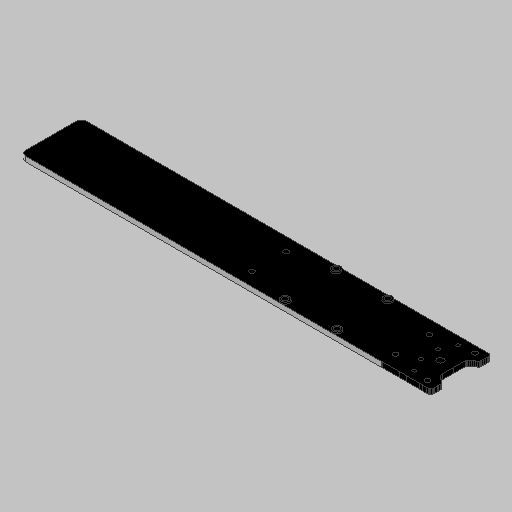
# Autodesk Inventor part: Part3
Saved by Autodesk Inventor 2025.2 (Build 292293000, 293)
## iProperties
Created: 2025-03-10
Part Number: Part3
Material: Generic
Document SubType Name: Modeling
Designer: joaki
Density: 1 g/cm^3
Appearance: Default
Author: joaki
Autodesk Inventor part; units mm, degrees
(part 1 of 5)
ref_plane "YZ Plane" through (0, 0, 0) normal (1, 0, 0) x (0, 1, 0)
ref_plane "XZ Plane" through (0, 0, 0) normal (0, 1, 0) x (-1, 0, 0)
ref_plane "XY Plane" through (0, 0, 0) normal (0, 0, 1) x (1, 0, 0)
sketch "Sketch1" plane through (0, 0, 0) normal (0, 1, 0) x (-1, 0, 0)
  arc A0 (-32.0458, 49.1475) -> (-32.3532, 49.036) centre (-31.3396, 46.7212) ccw
  arc A1 (-32.3532, 49.036) -> (-32.6918, 48.8703) centre (-30.5708, 44.9654) ccw
  arc A2 (-32.6918, 48.8703) -> (-33.0092, 48.6799) centre (-30.623, 45.0615) ccw
  arc A3 (-33.0092, 48.6799) -> (-33.2503, 48.4933) centre (-31.9001, 46.9981) ccw
  arc A4 (-33.2503, 48.4933) -> (-33.966, 47.6322) centre (-30.6139, 45.5739) ccw
  arc A5 (-33.966, 47.6322) -> (-35.7265, 44.7103) centre (138.8211, -58.464) ccw
  arc A6 (-35.7265, 44.7103) -> (-37.4503, 41.7415) centre (154.4036, -67.6751) ccw
  arc A7 (-37.4503, 41.7415) -> (-37.8104, 40.7786) centre (-34.6555, 40.1476) ccw
  arc A8 (-37.8104, 40.7786) -> (-37.8194, 40.2827) centre (-36.4462, 40.5057) ccw
  arc A9 (-37.8194, 40.2827) -> (-37.3843, 37.657) centre (368.8514, 106.3279) ccw
  arc A10 (-37.3843, 37.657) -> (-36.8416, 34.5948) centre (155.765, 70.3074) ccw
  arc A11 (-36.8416, 34.5948) -> (-36.1725, 31.0888) centre (296.5053, 96.4035) ccw
  arc A12 (-35.5034, 27.5915) -> (-36.1725, 31.0888) centre (-396.5345, -39.6615) ccw
  arc A13 (-34.9615, 24.557) -> (-35.5034, 27.5915) centre (-238.8908, -10.2959) ccw
  arc A14 (-34.5206, 21.9365) -> (-34.9615, 24.557) centre (-543.7583, -62.3998) ccw
  arc A15 (-34.5375, 21.5226) -> (-34.5206, 21.9365) centre (-35.5244, 21.7703) ccw
  arc A16 (-34.665, 21.2419) -> (-34.5375, 21.5226) centre (-35.3707, 21.7317) ccw
  arc A17 (-34.9963, 20.7996) -> (-34.665, 21.2419) centre (-40.9474, 25.6026) ccw
  arc A18 (-35.4254, 20.3066) -> (-34.9963, 20.7996) centre (-41.848, 26.3295) ccw
  arc A19 (-35.9077, 19.8249) -> (-35.4254, 20.3066) centre (-43.0211, 27.4297) ccw
  line L0 (-35.9077, 19.8249) -> (-37.1415, 18.6708)
  line L1 (-37.1415, 18.6708) -> (-50.9288, 18.6708)
  line L2 (-50.9288, 18.6708) -> (-64.716, 18.6708)
  line L3 (-64.716, 18.6708) -> (-65.4406, 17.9462)
  arc A20 (-65.4406, 17.9462) -> (-65.8665, 17.4366) centre (-62.8082, 15.3139) ccw
  arc A21 (-65.8665, 17.4366) -> (-66.0686, 16.973) centre (-64.7983, 16.6952) ccw
  arc A22 (-66.0686, 16.973) -> (-66.1492, 16.2892) centre (-62.6302, 16.221) ccw
  arc A23 (-66.1492, 16.2892) -> (-66.1652, 14.6332) centre (19.2549, 14.6332) ccw
  arc A24 (-66.1652, 14.6332) -> (-66.0935, 12.6637) centre (-39.0795, 14.6332) ccw
  arc A25 (-66.0935, 12.6637) -> (-65.8047, 11.6707) centre (-63.6234, 12.8438) ccw
  arc A26 (-65.8047, 11.6707) -> (-65.1416, 10.9064) centre (-63.7738, 12.7629) ccw
  arc A27 (-65.1416, 10.9064) -> (-63.6042, 9.8709) centre (-52.1239, 28.5747) ccw
  arc A28 (-62.9662, 9.4495) -> (-63.6042, 9.8709) centre (-69.6262, 0.0598) ccw
  arc A29 (-62.3849, 9.0034) -> (-62.9662, 9.4495) centre (-68.5849, 1.5279) ccw
  arc A30 (-61.9232, 8.5909) -> (-62.3849, 9.0034) centre (-67.7613, 2.5209) ccw
  arc A31 (-61.7221, 8.31) -> (-61.9232, 8.5909) centre (-62.5797, 7.9083) ccw
  arc A32 (-61.4522, 7.1095) -> (-61.7221, 8.31) centre (-64.311, 7.0975) ccw
  arc A33 (-61.449, 0.3443) -> (-61.4522, 7.1095) centre (-966.3811, 3.2944) ccw
  arc A34 (-61.4895, -6.5686) -> (-61.449, 0.3443) centre (-1389.8333, 4.6747) ccw
  arc A35 (-61.7732, -7.3571) -> (-61.4895, -6.5686) centre (-62.7573, -6.5578) ccw
  arc A36 (-61.9835, -7.5631) -> (-61.7732, -7.3571) centre (-62.7825, -6.5373) ccw
  arc A37 (-62.517, -7.9679) -> (-61.9835, -7.5631) centre (-78.0906, 13.1153) ccw
  arc A38 (-63.1677, -8.4333) -> (-62.517, -7.9679) centre (-77.9814, 12.9674) ccw
  arc A39 (-63.8815, -8.9144) -> (-63.1677, -8.4333) centre (-83.0238, 20.252) ccw
  arc A40 (-63.8815, -8.9144) -> (-64.619, -9.4313) centre (-55.7825, -21.2545) ccw
  arc A41 (-64.619, -9.4313) -> (-65.2474, -9.9433) centre (-58.8117, -17.2015) ccw
  arc A42 (-65.2474, -9.9433) -> (-65.7227, -10.4032) centre (-60.2081, -15.6266) ccw
  arc A43 (-65.7227, -10.4032) -> (-65.9266, -10.7277) centre (-65.0137, -11.0748) ccw
  arc A44 (-65.9266, -10.7277) -> (-66.0195, -11.1058) centre (-64.4333, -11.2955) ccw
  arc A45 (-66.0195, -11.1058) -> (-66.0951, -11.8637) centre (-46.7413, -13.4108) ccw
  arc A46 (-66.0951, -11.8637) -> (-66.1477, -12.7646) centre (-45.1165, -13.5407) ccw
  arc A47 (-66.1477, -12.7646) -> (-66.1652, -13.7133) centre (-40.4419, -13.7133) ccw
  arc A48 (-66.1652, -13.7133) -> (-66.1479, -15.1982) centre (-2.5179, -13.7133) ccw
  arc A49 (-66.1479, -15.1982) -> (-66.0652, -15.8456) centre (-62.9983, -15.1247) ccw
  arc A50 (-66.0652, -15.8456) -> (-65.8627, -16.2951) centre (-64.8098, -15.5505) ccw
  arc A51 (-65.8627, -16.2951) -> (-65.4406, -16.7957) centre (-62.7118, -14.0669) ccw
  line L4 (-65.4406, -16.7957) -> (-64.716, -17.5203)
  line L5 (-64.716, -17.5203) -> (-50.9288, -17.5203)
  line L6 (-50.9288, -17.5203) -> (-37.1415, -17.5203)
  line L7 (-37.1415, -17.5203) -> (-35.9077, -18.6744)
  arc A52 (-35.4252, -19.1571) -> (-35.9077, -18.6744) centre (-42.8603, -26.1072) ccw
  arc A53 (-34.9953, -19.6532) -> (-35.4252, -19.1571) centre (-41.7875, -25.1044) ccw
  arc A54 (-34.6634, -20.0994) -> (-34.9953, -19.6532) centre (-40.8736, -24.3709) ccw
  arc A55 (-34.534, -20.386) -> (-34.6634, -20.0994) centre (-35.3938, -20.6018) ccw
  arc A56 (-34.5166, -20.8095) -> (-34.534, -20.386) centre (-35.5445, -20.6396) ccw
  arc A57 (-34.9565, -23.4263) -> (-34.5166, -20.8095) centre (-518.611, 59.2131) ccw
  arc A58 (-35.4987, -26.4597) -> (-34.9565, -23.4263) centre (-233.6422, 10.5217) ccw
  arc A59 (-36.1687, -29.953) -> (-35.4987, -26.4597) centre (-386.2783, 39.0092) ccw
  arc A60 (-36.1687, -29.953) -> (-36.8391, -33.4539) centre (295.6451, -95.311) ccw
  arc A61 (-36.8391, -33.4539) -> (-37.3829, -36.5116) centre (155.2464, -69.1902) ccw
  arc A62 (-37.3829, -36.5116) -> (-37.8189, -39.1335) centre (367.7622, -105.2425) ccw
  arc A63 (-37.8189, -39.1335) -> (-37.8101, -39.6288) centre (-36.4488, -39.3568) ccw
  arc A64 (-37.8101, -39.6288) -> (-37.4483, -40.5963) centre (-34.644, -38.9963) ccw
  arc A65 (-37.4483, -40.5963) -> (-35.7241, -43.5638) centre (152.0351, 67.5195) ccw
  arc A66 (-35.7241, -43.5638) -> (-33.963, -46.4834) centre (136.2507, 58.1811) ccw
  arc A67 (-33.963, -46.4834) -> (-33.2418, -47.3505) centre (-30.5803, -44.4034) ccw
  arc A68 (-33.2418, -47.3505) -> (-32.6079, -47.7609) centre (-31.6519, -45.59) ccw
  arc A69 (-32.6079, -47.7609) -> (-31.8115, -48.0026) centre (-31.2092, -44.5847) ccw
  arc A70 (-31.8115, -48.0026) -> (-30.9596, -48.0512) centre (-31.1794, -44.4153) ccw
  arc A71 (-30.9596, -48.0512) -> (-30.1622, -47.8931) centre (-31.1413, -45.045) ccw
  arc A72 (-30.1622, -47.8931) -> (-29.6876, -47.6705) centre (-30.9566, -45.5823) ccw
  arc A73 (-29.6876, -47.6705) -> (-28.8553, -47.1427) centre (-43.1692, -25.4874) ccw
  arc A74 (-28.8553, -47.1427) -> (-27.8997, -46.4828) centre (-44.5769, -23.3578) ccw
  arc A75 (-27.8997, -46.4828) -> (-26.9312, -45.7575) centre (-47.5504, -19.2347) ccw
  arc A76 (-25.9779, -45.0187) -> (-26.9312, -45.7575) centre (214.0205, -355.696) ccw
  arc A77 (-25.0682, -44.3185) -> (-25.9779, -45.0187) centre (171.1636, -300.2176) ccw
  arc A78 (-24.2959, -43.7282) -> (-25.0682, -44.3185) centre (161.6381, -287.7955) ccw
  arc A79 (-23.908, -43.4391) -> (-24.2959, -43.7282) centre (-10.4312, -61.9278) ccw
  arc A80 (-23.908, -43.4391) -> (-23.635, -43.2176) centre (-25.9078, -40.6956) ccw
  arc A81 (-23.635, -43.2176) -> (-23.3603, -42.9495) centre (-26.861, -39.6379) ccw
  arc A82 (-23.3603, -42.9495) -> (-23.1231, -42.6775) centre (-26.5893, -39.8949) ccw
  arc A83 (-23.1231, -42.6775) -> (-22.97, -42.4476) centre (-24.338, -41.7022) ccw
  arc A84 (-22.97, -42.4476) -> (-22.8216, -42.0561) centre (-24.3206, -41.7117) ccw
  arc A85 (-22.8216, -42.0561) -> (-22.3963, -40.1768) centre (-302.2777, 22.1631) ccw
  arc A86 (-22.3963, -40.1768) -> (-21.92, -37.963) centre (-175.4238, -6.0918) ccw
  arc A87 (-21.92, -37.963) -> (-21.4078, -35.4342) centre (-280.1237, 15.6466) ccw
  arc A88 (-20.7015, -31.9464) -> (-21.4078, -35.4342) centre (334.9822, -105.7994) ccw
  arc A89 (-20.2507, -30.0187) -> (-20.7015, -31.9464) centre (18.1429, -40.0119) ccw
  arc A90 (-19.8825, -28.8183) -> (-20.2507, -30.0187) centre (-6.1073, -33.7001) ccw
  arc A91 (-19.5036, -28.1181) -> (-19.8825, -28.8183) centre (-17.4599, -29.6768) ccw
  arc A92 (-18.8502, -27.5305) -> (-19.5036, -28.1181) centre (-17.6228, -29.5526) ccw
  arc A93 (-17.2291, -26.6008) -> (-18.8502, -27.5305) centre (0.7057, -59.7481) ccw
  arc A94 (-14.6233, -25.2496) -> (-17.2291, -26.6008) centre (22.466, -99.9656) ccw
  arc A95 (-9.9894, -22.9703) -> (-14.6233, -25.2496) centre (300.6104, -660.2864) ccw
  line L8 (-9.9894, -22.9703) -> (-1.0955, -18.6358)
  line L9 (-1.0955, -18.6358) -> (8.0762, -18.6358)
  line L10 (8.0762, -18.6358) -> (17.2479, -18.6358)
  line L11 (17.2479, -18.6358) -> (24.8084, -22.3417)
  line L12 (24.8084, -22.3417) -> (32.3689, -26.0476)
  line L13 (32.3689, -26.0476) -> (35.2196, -26.2019)
  arc A96 (36.4236, -26.2887) -> (35.2196, -26.2019) centre (33.3912, -59.9686) ccw
  arc A97 (37.4686, -26.4112) -> (36.4236, -26.2887) centre (34.6684, -45.7838) ccw
  arc A98 (38.3015, -26.5549) -> (37.4686, -26.4112) centre (35.2575, -41.7081) ccw
  arc A99 (38.7351, -26.7101) -> (38.3015, -26.5549) centre (37.9884, -28.1134) ccw
  arc A100 (39.4307, -27.1904) -> (38.7351, -26.7101) centre (37.0105, -29.951) ccw
  arc A101 (40.7715, -28.4019) -> (39.4307, -27.1904) centre (-0.28, -72.4878) ccw
  arc A102 (42.9941, -30.5084) -> (40.7715, -28.4019) centre (-77.6934, -155.6235) ccw
  arc A103 (47.6927, -35.0512) -> (42.9941, -30.5084) centre (-1940.1141, -2086.3727) ccw
  arc A104 (47.6927, -35.0512) -> (49.3423, -36.6259) centre (153.8346, 74.4823) ccw
  arc A105 (49.3423, -36.6259) -> (50.8491, -38.014) centre (117.4767, 35.8224) ccw
  arc A106 (50.8491, -38.014) -> (52.1319, -39.156) centre (136.8471, 57.2886) ccw
  arc A107 (52.1319, -39.156) -> (52.5832, -39.4642) centre (53.6168, -37.4655) ccw
  arc A108 (52.5832, -39.4642) -> (53.1272, -39.6477) centre (53.4552, -37.778) ccw
  arc A109 (53.1272, -39.6477) -> (54.1122, -39.7872) centre (55.7356, -24.7774) ccw
  arc A110 (54.1122, -39.7872) -> (55.5073, -39.9019) centre (57.0387, -12.7301) ccw
  arc A111 (55.5073, -39.9019) -> (57.4953, -39.9955) centre (61.5401, 67.1382) ccw
  arc A112 (57.4953, -39.9955) -> (60.1211, -40.0813) centre (67.2669, 218.8167) ccw
  arc A113 (60.1211, -40.0813) -> (61.2161, -40.0556) centre (60.4171, -29.3564) ccw
  arc A114 (61.2161, -40.0556) -> (61.9074, -39.9182) centre (60.9996, -37.1571) ccw
  arc A115 (61.9074, -39.9182) -> (62.553, -39.6178) centre (60.9627, -37.0446) ccw
  arc A116 (62.553, -39.6178) -> (63.401, -38.8666) centre (60.8065, -36.7919) ccw
  arc A117 (63.401, -38.8666) -> (63.8273, -37.9517) centre (61.7324, -37.5323) ccw
  arc A118 (63.8273, -37.9517) -> (63.945, -36.4888) centre (57.6795, -36.721) ccw
  arc A119 (63.945, -36.4888) -> (63.7828, -33.4743) centre (-26.3737, -39.836) ccw
  arc A120 (63.7828, -33.4743) -> (63.6405, -31.7408) centre (-11.7723, -38.8057) ccw
  arc A121 (63.6405, -31.7408) -> (63.4783, -30.3261) centre (29.4973, -34.9394) ccw
  arc A122 (63.4783, -30.3261) -> (63.3076, -29.2348) centre (36.4135, -34.0005) ccw
  arc A123 (63.3076, -29.2348) -> (63.1401, -28.7399) centre (61.5967, -29.538) ccw
  arc A124 (63.1401, -28.7399) -> (62.9109, -28.3877) centre (61.2637, -29.7102) ccw
  arc A125 (62.9109, -28.3877) -> (62.4619, -27.8552) centre (51.6154, -37.4562) ccw
  arc A126 (62.4619, -27.8552) -> (61.9144, -27.2663) centre (50.1465, -38.7565) ccw
  arc A127 (61.9144, -27.2663) -> (61.3334, -26.6988) centre (49.6638, -39.2277) ccw
  arc A128 (60.5066, -25.919) -> (61.3334, -26.6988) centre (123.3408, 39.8753) ccw
  arc A129 (58.9809, -24.4587) -> (60.5066, -25.919) centre (705.9023, 649.8816) ccw
  arc A130 (57.1984, -22.7446) -> (58.9809, -24.4587) centre (761.7671, 708.1167) ccw
  arc A131 (55.3602, -20.9685) -> (57.1984, -22.7446) centre (862.103, 812.1978) ccw
  arc A132 (52.2259, -17.8854) -> (55.3602, -20.9685) centre (249.3198, 179.3436) ccw
  arc A133 (51.1754, -16.6035) -> (52.2259, -17.8854) centre (58.1388, -11.9685) ccw
  arc A134 (50.865, -15.6332) -> (51.1754, -16.6035) centre (52.7225, -15.5738) ccw
  arc A135 (51.0545, -14.4999) -> (50.865, -15.6332) centre (53.7892, -15.5396) ccw
  arc A136 (51.0545, -14.4999) -> (51.1419, -14.2671) centre (23.7331, -4.1123) ccw
  arc A137 (51.1419, -14.2671) -> (51.224, -14.0421) centre (27.5582, -5.5295) ccw
  arc A138 (51.224, -14.0421) -> (51.2922, -13.8498) centre (29.2984, -6.1554) ccw
  arc A139 (51.2922, -13.8498) -> (51.3252, -13.7472) centre (49.285, -13.1476) ccw
  arc A140 (51.365, -13.6156) -> (51.3252, -13.7472) centre (60.1692, -16.3465) ccw
  arc A141 (51.573, -12.9453) -> (51.365, -13.6156) centre (2315.9891, -716.0608) ccw
  arc A142 (51.8163, -12.1627) -> (51.573, -12.9453) centre (1163.3252, -358.1505) ccw
  arc A143 (52.0949, -11.2683) -> (51.8163, -12.1627) centre (1946.7401, -602.0111) ccw
  line L14 (52.0949, -11.2683) -> (52.8121, -8.9683)
  line L15 (52.8121, -8.9683) -> (52.2058, -7.7241)
  arc A144 (52.2058, -7.7241) -> (51.6635, -6.7311) centre (41.2407, -13.0675) ccw
  arc A145 (51.6635, -6.7311) -> (51.1218, -5.9924) centre (47.1312, -9.4864) ccw
  arc A146 (51.1218, -5.9924) -> (50.6059, -5.522) centre (48.7795, -8.0432) ccw
  arc A147 (50.6059, -5.522) -> (50.145, -5.3705) centre (50.1383, -6.1675) ccw
  arc A148 (50.145, -5.3705) -> (43.9407, -5.3415) centre (43.0705, -856.1898) ccw
  arc A149 (43.9407, -5.3415) -> (39.5994, -5.3815) centre (43.724, -217.1659) ccw
  arc A150 (39.5994, -5.3815) -> (36.3061, -5.461) centre (46.5143, -360.4549) ccw
  arc A151 (36.3061, -5.461) -> (35.8057, -5.6497) centre (36.3297, -6.281) ccw
  arc A152 (35.558, -5.7744) -> (35.8057, -5.6497) centre (35.4116, -5.1748) ccw
  arc A153 (34.9808, -5.8969) -> (35.558, -5.7744) centre (33.2428, 3.7067) ccw
  arc A154 (34.2764, -6) -> (34.9808, -5.8969) centre (33.1015, 4.487) ccw
  arc A155 (33.5111, -6.065) -> (34.2764, -6) centre (32.685, 8.2054) ccw
  arc A156 (32.4764, -6.0996) -> (33.5111, -6.065) centre (32.2851, 15.1126) ccw
  arc A157 (31.7452, -6.0576) -> (32.4764, -6.0996) centre (32.4267, -0.5824) ccw
  arc A158 (31.1271, -5.9276) -> (31.7452, -6.0576) centre (32.2133, -2.2969) ccw
  arc A159 (30.4757, -5.6872) -> (31.1271, -5.9276) centre (32.7103, -0.6353) ccw
  arc A160 (29.3977, -5.1026) -> (30.4757, -5.6872) centre (33.5644, 1.2955) ccw
  arc A161 (28.4534, -4.3647) -> (29.3977, -5.1026) centre (33.2018, 0.7387) ccw
  arc A162 (27.6607, -3.4863) -> (28.4534, -4.3647) centre (33.0763, 0.6038) ccw
  arc A163 (27.0334, -2.4843) -> (27.6607, -3.4863) centre (33.0572, 0.5894) ccw
  arc A164 (26.5396, -1.0622) -> (27.0334, -2.4843) centre (31.9221, 0.0102) ccw
  arc A165 (26.3831, 0.5941) -> (26.5396, -1.0622) centre (34.5147, 0.5267) ccw
  arc A166 (26.5671, 2.2507) -> (26.3831, 0.5941) centre (34.5425, 0.5265) ccw
  arc A167 (27.0845, 3.6738) -> (26.5671, 2.2507) centre (32.0341, 1.0688) ccw
  arc A168 (28.6323, 5.6815) -> (27.0845, 3.6738) centre (33.6271, 0.2303) ccw
  arc A169 (30.6893, 6.9123) -> (28.6323, 5.6815) centre (32.6578, 1.2881) ccw
  arc A170 (33.1577, 7.2725) -> (30.6893, 6.9123) centre (32.851, 0.7362) ccw
  arc A171 (35.8933, 6.757) -> (33.1577, 7.2725) centre (32.6882, -2.7338) ccw
  arc A172 (35.8933, 6.757) -> (36.9859, 6.4742) centre (38.3889, 14.1469) ccw
  arc A173 (36.9859, 6.4742) -> (38.159, 6.3355) centre (38.6678, 15.6719) ccw
  arc A174 (38.159, 6.3355) -> (39.9552, 6.2908) centre (39.8146, 36.7178) ccw
  arc A175 (39.9552, 6.2908) -> (43.8542, 6.3232) centre (37.5142, 534.6254) ccw
  arc A176 (43.8542, 6.3232) -> (48.7398, 6.4156) centre (39.6116, 359.8817) ccw
  arc A177 (48.7398, 6.4156) -> (50.2651, 6.6515) centre (48.5834, 12.4744) ccw
  arc A178 (50.2651, 6.6515) -> (51.1907, 7.2688) centre (49.7543, 8.4203) ccw
  arc A179 (51.1907, 7.2688) -> (52.1571, 8.7212) centre (43.5036, 13.431) ccw
  arc A180 (52.1571, 8.7212) -> (52.5499, 9.6239) centre (47.2365, 11.3993) ccw
  arc A181 (52.5499, 9.6239) -> (52.6227, 10.3337) centre (51.0016, 10.1413) ccw
  arc A182 (52.6227, 10.3337) -> (52.4152, 11.3392) centre (46.6444, 9.6239) ccw
  arc A183 (52.4152, 11.3392) -> (51.4783, 14.4385) centre (-281.7439, -87.9814) ccw
  arc A184 (51.2325, 15.2819) -> (51.4783, 14.4385) centre (80.2248, 23.274) ccw
  arc A185 (51.0249, 16.0887) -> (51.2325, 15.2819) centre (74.6872, 21.7475) ccw
  arc A186 (50.872, 16.7746) -> (51.0249, 16.0887) centre (73.247, 21.4031) ccw
  arc A187 (50.8363, 17.123) -> (50.872, 16.7746) centre (52.5561, 17.123) ccw
  arc A188 (51.0918, 17.7651) -> (50.8363, 17.123) centre (51.771, 17.123) ccw
  arc A189 (53.4926, 20.2635) -> (51.0918, 17.7651) centre (205.2647, -127.9862) ccw
  arc A190 (56.6261, 23.3714) -> (53.4926, 20.2635) centre (153.1437, -77.0747) ccw
  arc A191 (60.8135, 27.3373) -> (56.6261, 23.3714) centre (333.2856, -264.5481) ccw
  arc A192 (60.8135, 27.3373) -> (62.3235, 28.8541) centre (40.8815, 48.6894) ccw
  arc A193 (62.3235, 28.8541) -> (63.0421, 29.919) centre (59.2273, 31.7184) ccw
  arc A194 (63.0421, 29.919) -> (63.4263, 31.1789) centre (58.9127, 31.8668) ccw
  arc A195 (63.4263, 31.1789) -> (63.7028, 33.4626) centre (26.4707, 36.8114) ccw
  arc A196 (63.7028, 33.4626) -> (63.9582, 37.0302) centre (-34.0311, 42.2531) ccw
  arc A197 (63.9582, 37.0302) -> (63.849, 38.8602) centre (55.8311, 37.4633) ccw
  arc A198 (63.849, 38.8602) -> (63.3668, 39.9957) centre (61.1735, 38.3941) ccw
  arc A199 (63.3668, 39.9957) -> (62.414, 40.8601) centre (60.7933, 38.1165) ccw
  arc A200 (62.414, 40.8601) -> (61.8342, 41.0953) centre (61.3365, 39.0361) ccw
  arc A201 (61.8342, 41.0953) -> (61.1017, 41.2035) centre (60.8719, 37.1135) ccw
  arc A202 (61.1017, 41.2035) -> (59.9241, 41.2202) centre (60.314, 27.1829) ccw
  arc A203 (59.9241, 41.2202) -> (57.4704, 41.1378) centre (65.842, -171.8141) ccw
  arc A204 (57.4704, 41.1378) -> (55.5063, 41.042) centre (61.5593, -62.8736) ccw
  arc A205 (55.5063, 41.042) -> (54.1024, 40.9251) centre (57.1519, 12.7905) ccw
  arc A206 (54.1024, 40.9251) -> (53.1017, 40.7855) centre (55.8755, 24.5666) ccw
  arc A207 (53.1017, 40.7855) -> (52.5672, 40.6064) centre (53.4115, 38.9736) ccw
  arc A208 (52.5672, 40.6064) -> (52.1247, 40.3041) centre (53.5784, 38.651) ccw
  arc A209 (52.1247, 40.3041) -> (50.8788, 39.1934) centre (132.7429, -51.3769) ccw
  arc A210 (50.8788, 39.1934) -> (49.4154, 37.8426) centre (114.8118, -31.5387) ccw
  arc A211 (49.4154, 37.8426) -> (47.8149, 36.311) centre (149.4087, -68.2436) ccw
  arc A212 (41.2887, 30.0137) -> (47.8149, 36.311) centre (-858.6722, 969.2196) ccw
  arc A213 (39.2102, 28.2968) -> (41.2887, 30.0137) centre (28.6179, 43.2371) ccw
  arc A214 (37.5524, 27.5863) -> (39.2102, 28.2968) centre (36.7292, 31.7963) ccw
  arc A215 (35.1804, 27.3533) -> (37.5524, 27.5863) centre (35.1464, 39.8908) ccw
  line L16 (35.1804, 27.3533) -> (32.7864, 27.3468)
  line L17 (32.7864, 27.3468) -> (28.9833, 25.518)
  arc A216 (28.9833, 25.518) -> (27.2409, 24.6769) centre (313.7924, -566.75) ccw
  arc A217 (27.2409, 24.6769) -> (25.1323, 23.6531) centre (641.4444, -1243.0058) ccw
  arc A218 (25.1323, 23.6531) -> (23.0084, 22.6175) centre (646.446, -1253.2841) ccw
  arc A219 (23.0084, 22.6175) -> (21.2141, 21.7377) centre (343.666, -633.6275) ccw
  line L18 (21.2141, 21.7377) -> (17.2479, 19.7863)
  line L19 (17.2479, 19.7863) -> (8.0762, 19.7863)
  line L20 (8.0762, 19.7863) -> (-1.0955, 19.7863)
  line L21 (-1.0955, 19.7863) -> (-4.5659, 21.4751)
  arc A220 (-5.902, 22.1392) -> (-4.5659, 21.4751) centre (34.4649, 101.6796) ccw
  arc A221 (-7.0411, 22.7361) -> (-5.902, 22.1392) centre (16.4453, 66.1734) ccw
  arc A222 (-8.0069, 23.2643) -> (-7.0411, 22.7361) centre (47.8168, 124.1941) ccw
  arc A223 (-8.1189, 23.3962) -> (-8.0069, 23.2643) centre (-7.8886, 23.4782) ccw
  arc A224 (-8.1189, 23.3962) -> (-8.1783, 23.4851) centre (-8.3249, 23.323) ccw
  arc A225 (-8.1783, 23.4851) -> (-8.2876, 23.5603) centre (-8.5137, 23.1142) ccw
  arc A226 (-8.2876, 23.5603) -> (-8.4273, 23.6112) centre (-8.5693, 23.0045) ccw
  arc A227 (-8.4273, 23.6112) -> (-8.5771, 23.6285) centre (-8.5771, 22.9713) ccw
  arc A228 (-9.2372, 23.7793) -> (-8.5771, 23.6285) centre (-8.5771, 25.149) ccw
  arc A229 (-13.8235, 26.0012) -> (-9.2372, 23.7793) centre (531.9885, 1146.7753) ccw
  arc A230 (-18.2781, 28.1877) -> (-13.8235, 26.0012) centre (335.7059, 743.7276) ccw
  arc A231 (-19.1317, 28.7685) -> (-18.2781, 28.1877) centre (-16.615, 31.5494) ccw
  arc A232 (-19.695, 29.5249) -> (-19.1317, 28.7685) centre (-17.4997, 30.5719) ccw
  arc A233 (-20.1509, 30.7218) -> (-19.695, 29.5249) centre (-12.5561, 32.9295) ccw
  arc A234 (-20.6455, 32.7223) -> (-20.1509, 30.7218) centre (4.2642, 37.8192) ccw
  arc A235 (-21.4206, 36.6425) -> (-20.6455, 32.7223) centre (275.316, 93.281) ccw
  arc A236 (-21.4206, 36.6425) -> (-21.8747, 38.97) centre (-307.8728, -18.0332) ccw
  arc A237 (-21.8747, 38.97) -> (-22.2996, 41.0397) centre (-202.368, 2.9952) ccw
  arc A238 (-22.2996, 41.0397) -> (-22.6736, 42.7815) centre (-284.8038, -14.4217) ccw
  arc A239 (-22.6736, 42.7815) -> (-22.8182, 43.2575) centre (-25.7124, 42.1183) ccw
  arc A240 (-22.8182, 43.2575) -> (-23.2826, 43.9066) centre (-24.343, 42.6574) ccw
  arc A241 (-23.2826, 43.9066) -> (-25.7594, 45.9749) centre (-152.9824, -108.8932) ccw
  arc A242 (-25.7594, 45.9749) -> (-28.187, 47.9094) centre (-92.0276, -34.6932) ccw
  arc A243 (-28.187, 47.9094) -> (-29.5851, 48.8165) centre (-34.3725, 39.9061) ccw
  arc A244 (-29.5851, 48.8165) -> (-30.2009, 49.0825) centre (-31.4513, 45.3431) ccw
  arc A245 (-30.2009, 49.0825) -> (-30.8318, 49.2291) centre (-31.2895, 45.827) ccw
  arc A246 (-30.8318, 49.2291) -> (-31.4544, 49.251) centre (-31.2541, 46.0897) ccw
  arc A247 (-31.4544, 49.251) -> (-32.0458, 49.1475) centre (-31.2815, 46.5217) ccw
  arc A248 (-24.6295, 44.6303) -> (-27.2318, 46.6198) centre (-1153.7592, -1429.6204) ccw
  arc A249 (-23.9597, 44.0911) -> (-24.6295, 44.6303) centre (-35.3885, 30.5827) ccw
  arc A250 (-23.6158, 43.7396) -> (-23.9597, 44.0911) centre (-25.6524, 42.0904) ccw
  arc A251 (-23.3497, 43.3353) -> (-23.6158, 43.7396) centre (-25.5277, 42.1914) ccw
  arc A252 (-23.2124, 42.9637) -> (-23.3497, 43.3353) centre (-24.7051, 42.6234) ccw
  arc A253 (-22.8589, 41.3832) -> (-23.2124, 42.9637) centre (-216.3335, -1.0528) ccw
  arc A254 (-22.4639, 39.5116) -> (-22.8589, 41.3832) centre (-141.2085, 15.4249) ccw
  arc A255 (-22.0448, 37.3861) -> (-22.4639, 39.5116) centre (-217.395, -0.029) ccw
  arc A256 (-22.0448, 37.3861) -> (-21.1773, 32.913) centre (944.0764, 222.4265) ccw
  arc A257 (-21.1773, 32.913) -> (-20.788, 31.1801) centre (10.9276, 39.2163) ccw
  arc A258 (-20.788, 31.1801) -> (-20.4506, 30.16) centre (-13.4673, 33.0351) ccw
  arc A259 (-20.4506, 30.16) -> (-19.9972, 29.3053) centre (-15.84, 32.0582) ccw
  arc A260 (-19.9972, 29.3053) -> (-19.4748, 28.7522) centre (-18.143, 30.5332) ccw
  arc A261 (-19.4748, 28.7522) -> (-18.5177, 28.1127) centre (-12.9792, 37.4385) ccw
  arc A262 (-18.5177, 28.1127) -> (-16.9446, 27.2426) centre (-3.56, 53.299) ccw
  arc A263 (-16.9446, 27.2426) -> (-14.1095, 25.8087) centre (98.6023, 252.1828) ccw
  arc A264 (-12.0323, 24.7642) -> (-14.1095, 25.8087) centre (-144.6863, -236.4456) ccw
  arc A265 (-10.2032, 23.8221) -> (-12.0323, 24.7642) centre (-93.5253, -135.7035) ccw
  arc A266 (-8.6618, 23.0111) -> (-10.2032, 23.8221) centre (-144.065, -232.4641) ccw
  arc A267 (-8.2957, 22.7721) -> (-8.6618, 23.0111) centre (-9.7891, 20.8842) ccw
  arc A268 (-8.2957, 22.7721) -> (-8.0891, 22.6255) centre (-6.787, 24.6795) ccw
  arc A269 (-8.0891, 22.6255) -> (-7.8689, 22.5016) centre (-6.7999, 24.6592) ccw
  arc A270 (-7.8689, 22.5016) -> (-7.6663, 22.4146) centre (-6.9678, 24.3202) ccw
  arc A271 (-7.6663, 22.4146) -> (-7.5227, 22.3891) centre (-7.5227, 22.8063) ccw
  arc A272 (-7.3202, 22.3478) -> (-7.5227, 22.3891) centre (-7.5227, 21.8714) ccw
  arc A273 (-6.4013, 21.9522) -> (-7.3202, 22.3478) centre (-50.8568, -80.0366) ccw
  arc A274 (-5.3284, 21.4717) -> (-6.4013, 21.9522) centre (-29.9117, -31.985) ccw
  arc A275 (-4.1106, 20.9018) -> (-5.3284, 21.4717) centre (-47.3029, -69.8025) ccw
  line L22 (-4.1106, 20.9018) -> (-0.9872, 19.4145)
  line L23 (-0.9872, 19.4145) -> (8.0456, 19.4145)
  line L24 (8.0456, 19.4145) -> (17.0783, 19.4145)
  line L25 (17.0783, 19.4145) -> (20.8814, 21.2433)
  arc A276 (20.8814, 21.2433) -> (22.6238, 22.083) centre (-484.0773, 1071.3158) ccw
  arc A277 (22.6238, 22.083) -> (24.7324, 23.1025) centre (-1060.8925, 2265.7293) ccw
  arc A278 (24.7324, 23.1025) -> (26.8564, 24.1319) centre (-1069.3377, 2283.1714) ccw
  arc A279 (26.8564, 24.1319) -> (28.6506, 25.0043) centre (-535.7997, 1183.6537) ccw
  line L26 (28.6506, 25.0043) -> (32.6168, 26.9364)
  line L27 (32.6168, 26.9364) -> (35.4675, 27.0905)
  arc A280 (35.4675, 27.0905) -> (36.762, 27.1823) centre (33.3768, 65.7674) ccw
  arc A281 (36.762, 27.1823) -> (37.7902, 27.3064) centre (35.3738, 43.0055) ccw
  arc A282 (37.7902, 27.3064) -> (38.5752, 27.459) centre (36.2402, 37.3763) ccw
  arc A283 (38.5752, 27.459) -> (39.0671, 27.6446) centre (38.1092, 29.4382) ccw
  arc A284 (39.0671, 27.6446) -> (39.5441, 27.9774) centre (37.9108, 29.8097) ccw
  arc A285 (39.5441, 27.9774) -> (41.0144, 29.3026) centre (-80.191, 162.3059) ccw
  arc A286 (41.0144, 29.3026) -> (42.7403, 30.9043) centre (-46.4927, 125.3275) ccw
  arc A287 (42.7403, 30.9043) -> (44.6445, 32.7273) centre (-97.274, 179.0628) ccw
  arc A288 (49.183, 37.1068) -> (44.6445, 32.7273) centre (920.7182, -870.6146) ccw
  arc A289 (51.3557, 39.1139) -> (49.183, 37.1068) centre (102.3641, -18.2825) ccw
  arc A290 (52.6879, 40.2169) -> (51.3557, 39.1139) centre (67.7812, 20.6314) ccw
  arc A291 (53.4652, 40.5662) -> (52.6879, 40.2169) centre (53.809, 38.7621) ccw
  arc A292 (53.9251, 40.6276) -> (53.4652, 40.5662) centre (54.2464, 36.4668) ccw
  arc A293 (55.0648, 40.7097) -> (53.9251, 40.6276) centre (62.3734, -68.7941) ccw
  arc A294 (56.426, 40.7914) -> (55.0648, 40.7097) centre (61.87, -61.2525) ccw
  arc A295 (57.9032, 40.8624) -> (56.426, 40.7914) centre (63.9553, -100.343) ccw
  arc A296 (60.2699, 40.951) -> (57.9032, 40.8624) centre (67.2345, -176.8584) ccw
  arc A297 (61.2117, 40.9238) -> (60.2699, 40.951) centre (60.5177, 33.2008) ccw
  arc A298 (61.7943, 40.78) -> (61.2117, 40.9238) centre (61.0348, 38.9552) ccw
  arc A299 (62.3323, 40.4645) -> (61.7943, 40.78) centre (60.9108, 38.6572) ccw
  arc A300 (63.0608, 39.6824) -> (62.3323, 40.4645) centre (60.1827, 37.7316) ccw
  arc A301 (63.4137, 38.7986) -> (63.0608, 39.6824) centre (61.2209, 38.4353) ccw
  arc A302 (63.4931, 37.4258) -> (63.4137, 38.7986) centre (57.0278, 37.7406) ccw
  arc A303 (63.3114, 34.5548) -> (63.4931, 37.4258) centre (-35.2641, 42.2347) ccw
  arc A304 (63.0404, 31.6852) -> (63.3114, 34.5548) centre (-24.2415, 41.376) ccw
  arc A305 (62.7285, 30.2629) -> (63.0404, 31.6852) centre (56.1559, 32.4496) ccw
  arc A306 (62.1894, 29.2632) -> (62.7285, 30.2629) centre (59.6061, 31.3017) ccw
  arc A307 (61.2015, 28.2131) -> (62.1894, 29.2632) centre (55.6611, 34.4147) ccw
  arc A308 (61.2015, 28.2131) -> (60.5391, 27.603) centre (81.0051, 6.0463) ccw
  arc A309 (60.5391, 27.603) -> (58.9998, 26.1371) centre (529.6146, -466.4717) ccw
  arc A310 (58.9998, 26.1371) -> (57.172, 24.3841) centre (508.9651, -444.8584) ccw
  arc A311 (57.172, 24.3841) -> (55.2084, 22.4876) centre (667.1745, -609.179) ccw
  arc A312 (55.2084, 22.4876) -> (51.4074, 18.741) centre (270.2225, -199.4484) ccw
  arc A313 (51.4074, 18.741) -> (50.5853, 17.4879) centre (54.0351, 16.1207) ccw
  arc A314 (50.5853, 17.4879) -> (50.503, 16.1693) centre (52.5675, 16.7024) ccw
  arc A315 (50.503, 16.1693) -> (51.4316, 12.9575) centre (106.7705, 30.6979) ccw
  arc A316 (52.0487, 10.8827) -> (51.4316, 12.9575) centre (2.6597, -2.6776) ccw
  arc A317 (52.1512, 9.8856) -> (52.0487, 10.8827) centre (49.1159, 10.0775) ccw
  arc A318 (51.8997, 9.0474) -> (52.1512, 9.8856) centre (50.2221, 10.0076) ccw
  arc A319 (51.1073, 7.8259) -> (51.8997, 9.0474) centre (40.5312, 15.5545) ccw
  line L28 (51.1073, 7.8259) -> (50.3374, 6.7724)
  line L29 (50.3374, 6.7724) -> (43.5524, 6.7724)
  arc A320 (39.8156, 6.787) -> (43.5524, 6.7724) centre (43.5525, 484.6336) ccw
  arc A321 (37.8327, 6.8468) -> (39.8156, 6.787) centre (40.1627, 51.1676) ccw
  arc A322 (36.598, 6.9626) -> (37.8327, 6.8468) centre (38.6272, 21.9602) ccw
  arc A323 (35.8076, 7.1795) -> (36.598, 6.9626) centre (37.0113, 10.0171) ccw
  arc A324 (35.8076, 7.1795) -> (34.5626, 7.5186) centre (33.9399, 2.7764) ccw
  arc A325 (34.5626, 7.5186) -> (32.9984, 7.603) centre (33.2301, -2.6289) ccw
  arc A326 (32.9984, 7.603) -> (31.4161, 7.4463) centre (33.2352, -2.8538) ccw
  arc A327 (31.4161, 7.4463) -> (30.1113, 7.0505) centre (32.4088, 1.8255) ccw
  arc A328 (30.1113, 7.0505) -> (27.0346, 4.4487) centre (32.9692, 0.5508) ccw
  arc A329 (27.0346, 4.4487) -> (25.8897, 0.6058) centre (32.8637, 0.6201) ccw
  arc A330 (25.8897, 0.6058) -> (27.0473, -3.2592) centre (32.9695, 0.6204) ccw
  arc A331 (27.0473, -3.2592) -> (30.1379, -5.9131) centre (33.1838, 0.7607) ccw
  arc A332 (30.1379, -5.9131) -> (31.4238, -6.3153) centre (32.3812, -0.9978) ccw
  arc A333 (31.4238, -6.3153) -> (32.9951, -6.4727) centre (33.2131, 3.6221) ccw
  arc A334 (32.9951, -6.4727) -> (34.5562, -6.3835) centre (33.2099, 3.475) ccw
  arc A335 (34.5562, -6.3835) -> (35.8076, -6.0355) centre (33.906, -1.6225) ccw
  arc A336 (36.5972, -5.8141) -> (35.8076, -6.0355) centre (37.026, -8.8631) ccw
  arc A337 (37.8105, -5.6965) -> (36.5972, -5.8141) centre (38.5699, -19.8407) ccw
  arc A338 (39.7677, -5.6364) -> (37.8105, -5.6965) centre (40.0982, -48.3051) ccw
  arc A339 (43.5108, -5.6219) -> (39.7677, -5.6364) centre (43.5106, -488.7307) ccw
  arc A340 (48.6396, -5.6495) -> (43.5108, -5.6219) centre (43.5104, -481.9367) ccw
  arc A341 (50.092, -5.8454) -> (48.6396, -5.6495) centre (48.5755, -11.6055) ccw
  arc A342 (50.9531, -6.4169) -> (50.092, -5.8454) centre (49.6841, -7.3946) ccw
  arc A343 (51.8428, -7.8155) -> (50.9531, -6.4169) centre (43.6455, -12.0474) ccw
  line L30 (51.8428, -7.8155) -> (52.3994, -8.8937)
  line L31 (52.3994, -8.8937) -> (51.6087, -11.162)
  arc A344 (51.6087, -11.162) -> (51.0773, -12.7246) centre (154.1462, -46.903) ccw
  arc A345 (51.0773, -12.7246) -> (50.7858, -13.7001) centre (67.2816, -18.098) ccw
  arc A346 (50.7858, -13.7001) -> (50.5933, -14.5552) centre (61.6322, -16.5918) ccw
  arc A347 (50.5933, -14.5552) -> (50.4189, -15.6248) centre (76.1534, -19.271) ccw
  arc A348 (50.4189, -15.6248) -> (50.5367, -16.4487) centre (51.8958, -15.834) ccw
  arc A349 (50.5367, -16.4487) -> (51.1002, -17.3068) centre (53.5408, -15.09) ccw
  arc A350 (51.1002, -17.3068) -> (52.5304, -18.7828) centre (74.698, 4.1275) ccw
  arc A351 (52.5304, -18.7828) -> (58.6939, -24.735) centre (3130.1027, 3161.8952) ccw
  arc A352 (60.2424, -26.2602) -> (58.6939, -24.735) centre (-10.9202, -96.9609) ccw
  arc A353 (61.572, -27.6413) -> (60.2424, -26.2602) centre (17.0817, -69.1408) ccw
  arc A354 (62.6596, -28.8281) -> (61.572, -27.6413) centre (-5.1158, -89.8461) ccw
  arc A355 (62.8559, -29.1969) -> (62.6596, -28.8281) centre (62.0166, -29.407) ccw
  arc A356 (62.9287, -29.5929) -> (62.8559, -29.1969) centre (59.7754, -29.9681) ccw
  arc A357 (63.0563, -30.7085) -> (62.9287, -29.5929) centre (-60.8478, -44.3194) ccw
  arc A358 (63.1942, -32.0414) -> (63.0563, -30.7085) centre (-42.0314, -42.2525) ccw
  arc A359 (63.3296, -33.5089) -> (63.1942, -32.0414) centre (-90.5574, -46.9617) ccw
  arc A360 (63.5179, -36.2184) -> (63.3296, -33.5089) centre (-12.6809, -40.1538) ccw
  arc A361 (63.4356, -37.6047) -> (63.5179, -36.2184) centre (57.2533, -36.542) ccw
  arc A362 (63.0708, -38.5174) -> (63.4356, -37.6047) centre (61.1119, -37.2052) ccw
  arc A363 (62.331, -39.318) -> (63.0708, -38.5174) centre (60.1511, -36.5616) ccw
  arc A364 (61.779, -39.6392) -> (62.331, -39.318) centre (60.933, -37.5504) ccw
  arc A365 (61.172, -39.7829) -> (61.779, -39.6392) centre (61.0073, -37.7338) ccw
  arc A366 (60.1701, -39.806) -> (61.172, -39.7829) centre (60.4691, -31.0354) ccw
  arc A367 (57.5292, -39.7039) -> (60.1701, -39.806) centre (69.9833, 248.0478) ccw
  arc A368 (55.7752, -39.6089) -> (57.5292, -39.7039) centre (61.0255, 41.0787) ccw
  arc A369 (54.3624, -39.4879) -> (55.7752, -39.6089) centre (58.026, -5.0177) ccw
  arc A370 (53.2778, -39.3515) -> (54.3624, -39.4879) centre (57.3738, -11.1536) ccw
  arc A371 (52.8194, -39.2033) -> (53.2778, -39.3515) centre (53.4843, -37.9298) ccw
  arc A372 (52.4203, -38.9275) -> (52.8194, -39.2033) centre (53.7294, -37.4603) ccw
  arc A373 (51.1074, -37.7443) -> (52.4203, -38.9275) centre (171.0848, 94.068) ccw
  arc A374 (49.5687, -36.3191) -> (51.1074, -37.7443) centre (132.6385, 51.8295) ccw
  arc A375 (47.8617, -34.6907) -> (49.5687, -36.3191) centre (182.3635, 104.5946) ccw
  arc A376 (47.8617, -34.6907) -> (43.2688, -30.2663) centre (-1782.7173, -1930.371) ccw
  arc A377 (43.2688, -30.2663) -> (41.045, -28.1667) centre (-76.8371, -155.2473) ccw
  arc A378 (41.045, -28.1667) -> (39.6926, -26.9489) centre (-0.7095, -73.1794) ccw
  arc A379 (39.6926, -26.9489) -> (38.9824, -26.4542) centre (37.0919, -29.9248) ccw
  arc A380 (38.9824, -26.4542) -> (38.5426, -26.2925) centre (38.2144, -27.8641) ccw
  arc A381 (38.5426, -26.2925) -> (37.7333, -26.1493) centre (35.8155, -39.3507) ccw
  arc A382 (37.7333, -26.1493) -> (36.6987, -26.0292) centre (35.1258, -44.0985) ccw
  arc A383 (36.6987, -26.0292) -> (35.4675, -25.9435) centre (33.6126, -61.4829) ccw
  line L32 (35.4675, -25.9435) -> (32.6168, -25.7948)
  line L33 (32.6168, -25.7948) -> (24.8459, -22.0294)
  line L34 (24.8459, -22.0294) -> (17.075, -18.264)
  line L35 (17.075, -18.264) -> (8.0416, -18.264)
  line L36 (8.0416, -18.264) -> (-0.9918, -18.264)
  line L37 (-0.9918, -18.264) -> (-9.9588, -22.6088)
  arc A384 (-9.9588, -22.6088) -> (-13.4351, -24.3114) centre (189.4604, -434.1767) ccw
  arc A385 (-13.4351, -24.3114) -> (-16.4541, -25.8298) centre (104.6885, -262.93) ccw
  arc A386 (-16.4541, -25.8298) -> (-19.0256, -27.1522) centre (233.4789, -514.9974) ccw
  arc A387 (-19.0256, -27.1522) -> (-19.4783, -27.4727) centre (-18.1008, -28.939) ccw
  arc A388 (-19.4783, -27.4727) -> (-20.1116, -28.3126) centre (-17.3571, -29.7306) ccw
  arc A389 (-20.1116, -28.3126) -> (-20.5977, -29.5182) centre (-13.8288, -31.5469) ccw
  arc A390 (-20.5977, -29.5182) -> (-21.1026, -31.5222) centre (1.7093, -36.2038) ccw
  arc A391 (-21.1026, -31.5222) -> (-21.9043, -35.5672) centre (277.6817, -92.8407) ccw
  arc A392 (-22.7174, -39.7245) -> (-21.9043, -35.5672) centre (-511.1801, 57.9702) ccw
  arc A393 (-23.1456, -41.4944) -> (-22.7174, -39.7245) centre (-45.0714, -35.2536) ccw
  arc A394 (-23.5257, -42.4562) -> (-23.1456, -41.4944) centre (-28.1733, -40.0634) ccw
  arc A395 (-24.0171, -42.9901) -> (-23.5257, -42.4562) centre (-24.7413, -41.8303) ccw
  arc A396 (-24.0171, -42.9901) -> (-24.304, -43.1885) centre (-22.0422, -46.1523) ccw
  arc A397 (-24.304, -43.1885) -> (-25.0542, -43.7652) centre (56.9613, -149.6746) ccw
  arc A398 (-25.0542, -43.7652) -> (-25.9436, -44.4609) centre (45.9587, -135.4664) ccw
  arc A399 (-25.9436, -44.4609) -> (-26.9121, -45.2319) centre (77.8149, -175.7858) ccw
  arc A400 (-27.8869, -46.0031) -> (-26.9121, -45.2319) centre (-83.9176, 25.8316) ccw
  arc A401 (-28.796, -46.6995) -> (-27.8869, -46.0031) centre (-68.2808, 5.7843) ccw
  arc A402 (-29.5663, -47.2708) -> (-28.796, -46.6995) centre (-71.1667, 9.6202) ccw
  arc A403 (-29.8958, -47.4767) -> (-29.5663, -47.2708) centre (-31.1384, -45.1209) ccw
  arc A404 (-30.579, -47.7064) -> (-29.8958, -47.4767) centre (-30.9452, -45.4872) ccw
  arc A405 (-31.38, -47.7432) -> (-30.579, -47.7064) centre (-31.1348, -44.3382) ccw
  arc A406 (-32.1558, -47.5931) -> (-31.38, -47.7432) centre (-31.1412, -44.4276) ccw
  arc A407 (-32.7638, -47.2701) -> (-32.1558, -47.5931) centre (-31.563, -45.7435) ccw
  arc A408 (-33.5006, -46.4468) -> (-32.7638, -47.2701) centre (-30.7946, -44.7667) ccw
  arc A409 (-35.2422, -43.5758) -> (-33.5006, -46.4468) centre (104.2396, 39.0748) ccw
  arc A410 (-36.9138, -40.6825) -> (-35.2422, -43.5758) centre (95.0983, 33.6578) ccw
  arc A411 (-37.3261, -39.5707) -> (-36.9138, -40.6825) centre (-33.6252, -38.8306) ccw
  arc A412 (-37.3541, -39.1971) -> (-37.3261, -39.5707) centre (-35.8242, -39.2704) ccw
  arc A413 (-37.3056, -38.5298) -> (-37.3541, -39.1971) centre (-23.782, -39.8472) ccw
  arc A414 (-37.2096, -37.7514) -> (-37.3056, -38.5298) centre (-22.1023, -40.0109) ccw
  arc A415 (-37.0712, -36.9536) -> (-37.2096, -37.7514) centre (-20.054, -40.3172) ccw
  arc A416 (-37.0712, -36.9536) -> (-35.4855, -28.8679) centre (-2745.9567, 498.4883) ccw
  arc A417 (-35.4855, -28.8679) -> (-34.6127, -24.2087) centre (-368.1278, 35.8516) ccw
  arc A418 (-34.6127, -24.2087) -> (-34.0594, -21.0488) centre (-362.3965, 34.8192) ccw
  arc A419 (-34.0594, -21.0488) -> (-34.0855, -20.3742) centre (-35.6769, -20.7736) ccw
  arc A420 (-34.0855, -20.3742) -> (-34.2239, -20.0672) centre (-35.0102, -20.6063) ccw
  arc A421 (-34.2239, -20.0672) -> (-34.5803, -19.5857) centre (-41.0537, -24.7494) ccw
  arc A422 (-34.5803, -19.5857) -> (-35.0418, -19.0492) centre (-42.0413, -25.5371) ccw
  arc A423 (-35.0418, -19.0492) -> (-35.56, -18.5257) centre (-43.2558, -26.6628) ccw
  line L38 (-35.56, -18.5257) -> (-36.8852, -17.2724)
  line L39 (-36.8852, -17.2724) -> (-50.6689, -17.2724)
  line L40 (-50.6689, -17.2724) -> (-64.4526, -17.2724)
  line L41 (-64.4526, -17.2724) -> (-65.061, -16.664)
  arc A424 (-65.4007, -16.2293) -> (-65.061, -16.664) centre (-63.4588, -15.0618) ccw
  arc A425 (-65.5769, -15.7726) -> (-65.4007, -16.2293) centre (-64.1827, -15.497) ccw
  arc A426 (-65.6527, -15.0785) -> (-65.5769, -15.7726) centre (-61.6072, -14.9879) ccw
  arc A427 (-65.6695, -13.5857) -> (-65.6527, -15.0785) centre (0.9919, -13.5858) ccw
  arc A428 (-65.6576, -12.609) -> (-65.6695, -13.5857) centre (-25.3048, -13.5857) ccw
  arc A429 (-65.6219, -11.7175) -> (-65.6576, -12.609) centre (-37.5423, -13.2895) ccw
  arc A430 (-65.5713, -10.9747) -> (-65.6219, -11.7175) centre (-34.8766, -13.4387) ccw
  arc A431 (-65.5076, -10.694) -> (-65.5713, -10.9747) centre (-64.5655, -11.0555) ccw
  arc A432 (-65.3508, -10.4676) -> (-65.5076, -10.694) centre (-64.965, -10.9022) ccw
  arc A433 (-64.84, -10.0352) -> (-65.3508, -10.4676) centre (-55.9097, -21.101) ccw
  arc A434 (-64.1955, -9.5449) -> (-64.84, -10.0352) centre (-55.9796, -21.0144) ccw
  arc A435 (-63.4625, -9.0436) -> (-64.1955, -9.5449) centre (-52.3231, -26.1189) ccw
  arc A436 (-63.4625, -9.0436) -> (-62.7194, -8.5337) centre (-74.0157, 7.133) ccw
  arc A437 (-62.7194, -8.5337) -> (-62.0441, -8.0177) centre (-71.6619, 3.8685) ccw
  arc A438 (-62.0441, -8.0177) -> (-61.5015, -7.5553) centre (-70.8664, 2.8855) ccw
  arc A439 (-61.5015, -7.5553) -> (-61.2783, -7.2762) centre (-62.2275, -6.7459) ccw
  arc A440 (-61.2783, -7.2762) -> (-61.0492, -6.4223) centre (-62.8544, -6.3956) ccw
  arc A441 (-61.0492, -6.4223) -> (-60.9654, 0.2581) centre (-1550.8386, 15.5871) ccw
  arc A442 (-60.9654, 0.2581) -> (-60.9236, 6.7099) centre (-908.0714, 8.9745) ccw
  arc A443 (-60.9236, 6.7099) -> (-61.1189, 8.2094) centre (-66.66, 6.7252) ccw
  arc A444 (-61.1189, 8.2094) -> (-61.2933, 8.5231) centre (-61.8315, 8.0186) ccw
  arc A445 (-61.2933, 8.5231) -> (-61.7482, 8.9601) centre (-65.6996, 4.392) ccw
  arc A446 (-61.7482, 8.9601) -> (-62.3944, 9.469) centre (-67.5847, 2.2127) ccw
  arc A447 (-62.3944, 9.469) -> (-63.2287, 10.0344) centre (-73.9935, -6.7469) ccw
  arc A448 (-63.9959, 10.5482) -> (-63.2287, 10.0344) centre (-50.62, 29.6904) ccw
  arc A449 (-64.6821, 11.0538) -> (-63.9959, 10.5482) centre (-54.2806, 24.4517) ccw
  arc A450 (-65.2326, 11.5002) -> (-64.6821, 11.0538) centre (-54.4262, 24.2642) ccw
  arc A451 (-65.4277, 11.7416) -> (-65.2326, 11.5002) centre (-64.6974, 12.1325) ccw
  arc A452 (-65.5226, 12.0428) -> (-65.4277, 11.7416) centre (-64.6759, 12.144) ccw
  arc A453 (-65.5984, 12.7968) -> (-65.5226, 12.0428) centre (-45.4007, 14.4473) ccw
  arc A454 (-65.6518, 13.7068) -> (-65.5984, 12.7968) centre (-45.8287, 14.4123) ccw
  arc A455 (-65.6695, 14.6996) -> (-65.6518, 13.7068) centre (-37.7547, 14.6996) ccw
  arc A456 (-65.6529, 16.2301) -> (-65.6695, 14.6996) centre (5.2302, 14.6996) ccw
  arc A457 (-65.5766, 16.9262) -> (-65.6529, 16.2301) centre (-61.653, 16.1437) ccw
  arc A458 (-65.3966, 17.385) -> (-65.5766, 16.9262) centre (-64.2041, 16.6525) ccw
  arc A459 (-65.0451, 17.8304) -> (-65.3966, 17.385) centre (-63.3309, 16.1162) ccw
  arc A460 (-64.5589, 18.193) -> (-65.0451, 17.8304) centre (-63.556, 16.3412) ccw
  arc A461 (-64.0239, 18.3685) -> (-64.5589, 18.193) centre (-63.808, 16.8065) ccw
  arc A462 (-63.1356, 18.4303) -> (-64.0239, 18.3685) centre (-63.125, 11.8656) ccw
  arc A463 (-60.7691, 18.4215) -> (-63.1356, 18.4303) centre (-62.778, -202.3278) ccw
  arc A464 (-60.7691, 18.4215) -> (-58.7385, 18.4096) centre (-57.9435, 328.9101) ccw
  arc A465 (-58.7385, 18.4096) -> (-55.2197, 18.4031) centre (-52.3385, 2517.5096) ccw
  arc A466 (-55.2197, 18.4031) -> (-51.1447, 18.4014) centre (-52.0176, 2794.3409) ccw
  arc A467 (-51.1447, 18.4014) -> (-47.0055, 18.4056) centre (-52.0768, 2974.9348) ccw
  line L42 (-47.0055, 18.4056) -> (-36.8936, 18.4229)
  line L43 (-36.8936, 18.4229) -> (-35.6353, 19.6)
  arc A468 (-35.6353, 19.6) -> (-35.1373, 20.0934) centre (-43.9526, 28.4919) ccw
  arc A469 (-35.1373, 20.0934) -> (-34.6814, 20.6027) centre (-43.1051, 27.6844) ccw
  arc A470 (-34.6814, 20.6027) -> (-34.3185, 21.062) centre (-42.0508, 26.7981) ccw
  arc A471 (-34.3185, 21.062) -> (-34.155, 21.3608) centre (-35.3165, 21.8024) ccw
  arc A472 (-34.155, 21.3608) -> (-34.0925, 21.9108) centre (-35.2, 21.7581) ccw
  arc A473 (-34.0925, 21.9108) -> (-34.3851, 23.8804) centre (-128.168, 8.9384) ccw
  arc A474 (-34.3851, 23.8804) -> (-34.8694, 26.6835) centre (-141.7096, 6.781) ccw
  arc A475 (-34.8694, 26.6835) -> (-35.6931, 31.0151) centre (-613.1272, -81.0359) ccw
  arc A476 (-36.358, 34.5394) -> (-35.6931, 31.0151) centre (302.3293, 96.608) ccw
  arc A477 (-36.897, 37.617) -> (-36.358, 34.5394) centre (159.1934, 70.3768) ccw
  arc A478 (-37.3294, 40.2564) -> (-36.897, 37.617) centre (377.629, 106.8704) ccw
  arc A479 (-37.3199, 40.7523) -> (-37.3294, 40.2564) centre (-35.9485, 40.4781) ccw
  arc A480 (-36.924, 41.8255) -> (-37.3199, 40.7523) centre (-33.7107, 40.0305) ccw
  arc A481 (-35.3627, 44.5458) -> (-36.924, 41.8255) centre (81.271, -24.2006) ccw
  arc A482 (-33.7482, 47.2048) -> (-35.3627, 44.5458) centre (67.0361, -15.8102) ccw
  arc A483 (-32.9118, 48.2311) -> (-33.7482, 47.2048) centre (-29.2491, 44.3917) ccw
  arc A484 (-32.5186, 48.5551) -> (-32.9118, 48.2311) centre (-30.4845, 45.6867) ccw
  arc A485 (-32.1386, 48.7625) -> (-32.5186, 48.5551) centre (-31.448, 47.0454) ccw
  arc A486 (-31.7218, 48.8755) -> (-32.1386, 48.7625) centre (-31.452, 47.0554) ccw
  arc A487 (-31.2169, 48.9127) -> (-31.7218, 48.8755) centre (-31.2169, 45.4688) ccw
  arc A488 (-30.5636, 48.8127) -> (-31.2169, 48.9127) centre (-31.2169, 46.7292) ccw
  arc A489 (-29.8861, 48.5159) -> (-30.5636, 48.8127) centre (-31.5794, 45.5731) ccw
  arc A490 (-28.9487, 47.9048) -> (-29.8861, 48.5159) centre (-34.9132, 39.7789) ccw
  arc A491 (-27.2318, 46.6198) -> (-28.9487, 47.9048) centre (-96.9845, -44.7864) ccw
  arc A492 (-31.6051, 42.0004) -> (-32.6766, 40.7652) centre (-30.2038, 39.7024) ccw
  arc A493 (-32.6766, 40.7652) -> (-32.9015, 39.0721) centre (-29.7758, 39.5184) ccw
  arc A494 (-32.9015, 39.0721) -> (-32.2104, 37.4765) centre (-29.6376, 39.5382) ccw
  arc A495 (-32.2104, 37.4765) -> (-30.8214, 36.5118) centre (-29.8891, 39.3367) ccw
  arc A496 (-30.8214, 36.5118) -> (-29.0361, 36.4927) centre (-29.8986, 39.3077) ccw
  arc A497 (-29.0361, 36.4927) -> (-27.522, 37.5045) centre (-29.9634, 39.5189) ccw
  arc A498 (-27.522, 37.5045) -> (-26.8003, 39.1984) centre (-30.0294, 39.5734) ccw
  arc A499 (-26.8003, 39.1984) -> (-27.1276, 40.9885) centre (-29.8945, 39.5577) ccw
  arc A500 (-27.1276, 40.9885) -> (-27.9004, 41.8608) centre (-29.2379, 39.8973) ccw
  arc A501 (-27.9004, 41.8608) -> (-29.0781, 42.3728) centre (-29.836, 39.0193) ccw
  arc A502 (-29.0781, 42.3728) -> (-30.4064, 42.4285) centre (-29.8949, 38.7584) ccw
  arc A503 (-30.4064, 42.4285) -> (-31.6051, 42.0004) centre (-29.9739, 39.3255) ccw
  arc A504 (-27.8856, 41.4472) -> (-28.1543, 41.7108) centre (-29.2207, 40.3551) ccw
  arc A505 (-27.6133, 41.071) -> (-27.8856, 41.4472) centre (-30.9354, 38.9525) ccw
  arc A506 (-27.3781, 40.6503) -> (-27.6133, 41.071) centre (-31.1201, 38.8347) ccw
  arc A507 (-27.2213, 40.2477) -> (-27.3781, 40.6503) centre (-29.8007, 39.4749) ccw
  arc A508 (-27.1181, 39.2801) -> (-27.2213, 40.2477) centre (-29.757, 39.488) ccw
  arc A509 (-27.3711, 38.3388) -> (-27.1181, 39.2801) centre (-29.7747, 39.4894) ccw
  arc A510 (-27.957, 37.5246) -> (-27.3711, 38.3388) centre (-29.9351, 39.5662) ccw
  arc A511 (-28.812, 36.9245) -> (-27.957, 37.5246) centre (-30.2724, 39.9143) ccw
  arc A512 (-29.3983, 36.6669) -> (-28.812, 36.9245) centre (-32.2924, 44.0499) ccw
  arc A513 (-29.7721, 36.5903) -> (-29.3983, 36.6669) centre (-29.8068, 37.709) ccw
  arc A514 (-30.1587, 36.6417) -> (-29.7721, 36.5903) centre (-29.8093, 37.7899) ccw
  arc A515 (-30.8037, 36.8627) -> (-30.1587, 36.6417) centre (-27.2987, 46.0405) ccw
  arc A516 (-31.8839, 37.5426) -> (-30.8037, 36.8627) centre (-29.6405, 39.9084) ccw
  arc A517 (-32.5407, 38.5493) -> (-31.8839, 37.5426) centre (-30.0993, 39.4246) ccw
  arc A518 (-32.6724, 39.7425) -> (-32.5407, 38.5493) centre (-30.1073, 39.4217) ccw
  arc A519 (-32.2688, 40.9493) -> (-32.6724, 39.7425) centre (-29.4678, 39.3417) ccw
  arc A520 (-31.8371, 41.5383) -> (-32.2688, 40.9493) centre (-29.4222, 39.3156) ccw
  arc A521 (-31.3407, 41.9158) -> (-31.8371, 41.5383) centre (-30.5318, 40.3368) ccw
  arc A522 (-30.7007, 42.1255) -> (-31.3407, 41.9158) centre (-30.3579, 39.9975) ccw
  arc A523 (-29.8216, 42.2031) -> (-30.7007, 42.1255) centre (-29.7202, 36.0383) ccw
  arc A524 (-29.3376, 42.1782) -> (-29.8216, 42.2031) centre (-29.7628, 38.6301) ccw
  arc A525 (-28.8956, 42.0871) -> (-29.3376, 42.1782) centre (-29.6579, 39.5055) ccw
  arc A526 (-28.5001, 41.9306) -> (-28.8956, 42.0871) centre (-29.569, 39.8066) ccw
  arc A527 (-28.1543, 41.7108) -> (-28.5001, 41.9306) centre (-29.4213, 40.1001) ccw
  arc A528 (54.0494, 35.7849) -> (53.7412, 35.5023) centre (57.9512, 31.2201) ccw
  arc A529 (53.7412, 35.5023) -> (53.5343, 35.2639) centre (55.1388, 34.0807) ccw
  arc A530 (53.5343, 35.2639) -> (53.4548, 35.106) centre (53.9572, 34.9521) ccw
  arc A531 (53.4548, 35.106) -> (53.5011, 35.0413) centre (53.5027, 35.0913) ccw
  arc A532 (53.5011, 35.0413) -> (53.6195, 35.0519) centre (53.517, 35.5303) ccw
  arc A533 (53.6195, 35.0519) -> (53.7199, 35.0913) centre (53.5498, 35.3772) ccw
  arc A534 (53.7199, 35.0913) -> (53.787, 35.1523) centre (53.604, 35.286) ccw
  arc A535 (53.787, 35.1523) -> (53.8109, 35.2256) centre (53.6866, 35.2256) ccw
  arc A536 (53.8522, 35.326) -> (53.8109, 35.2256) centre (53.9535, 35.2256) ccw
  arc A537 (54.0369, 35.4965) -> (53.8522, 35.326) centre (55.8531, 33.3431) ccw
  arc A538 (54.2856, 35.6863) -> (54.0369, 35.4965) centre (56.1107, 33.0377) ccw
  arc A539 (54.5803, 35.8745) -> (54.2856, 35.6863) centre (57.1283, 31.5611) ccw
  arc A540 (55.8004, 36.2372) -> (54.5803, 35.8745) centre (55.9167, 33.6121) ccw
  arc A541 (57.0918, 36.0022) -> (55.8004, 36.2372) centre (55.931, 33.2893) ccw
  arc A542 (58.1349, 35.2371) -> (57.0918, 36.0022) centre (55.9691, 33.3783) ccw
  arc A543 (58.6681, 34.1256) -> (58.1349, 35.2371) centre (56.3284, 33.6867) ccw
  arc A544 (58.7402, 33.3623) -> (58.6681, 34.1256) centre (54.536, 33.3504) ccw
  arc A545 (58.6484, 32.7101) -> (58.7402, 33.3623) centre (56.4253, 33.3557) ccw
  arc A546 (58.3729, 32.0936) -> (58.6484, 32.7101) centre (56.2851, 33.3964) ccw
  arc A547 (57.8873, 31.4369) -> (58.3729, 32.0936) centre (53.9695, 34.8414) ccw
  arc A548 (57.4927, 31.042) -> (57.8873, 31.4369) centre (54.8592, 34.0683) ccw
  arc A549 (57.141, 30.8268) -> (57.4927, 31.042) centre (56.678, 31.9782) ccw
  arc A550 (56.7102, 30.7233) -> (57.141, 30.8268) centre (56.5749, 32.2347) ccw
  arc A551 (56.038, 30.6932) -> (56.7102, 30.7233) centre (56.038, 38.2289) ccw
  arc A552 (55.3767, 30.726) -> (56.038, 30.6932) centre (56.038, 37.3822) ccw
  arc A553 (54.9152, 30.8336) -> (55.3767, 30.726) centre (55.5574, 32.5446) ccw
  arc A554 (54.5147, 31.0513) -> (54.9152, 30.8336) centre (55.4936, 32.3748) ccw
  arc A555 (54.0567, 31.4369) -> (54.5147, 31.0513) centre (57.3469, 34.8803) ccw
  arc A556 (53.6203, 31.9033) -> (54.0567, 31.4369) centre (58.0039, 35.5679) ccw
  arc A557 (53.4145, 32.269) -> (53.6203, 31.9033) centre (54.5014, 32.6398) ccw
  arc A558 (53.3388, 32.7121) -> (53.4145, 32.269) centre (54.7534, 32.7259) ccw
  arc A559 (53.3588, 33.4823) -> (53.3388, 32.7121) centre (64.1438, 32.8168) ccw
  arc A560 (53.3588, 33.4823) -> (53.3762, 34.0151) centre (44.1675, 34.0494) ccw